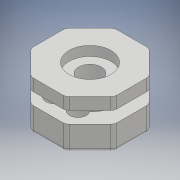
# Autodesk Inventor part: tendon anchor
Saved by Autodesk Inventor 2017 (Build 210142000, 142)
## iProperties
Created: 2018-09-01
Part Number: tendon anchor
Material: Generic
Document SubType Name: Modeling
Designer: jakub.tomczynski
Density: 1 g/cm^3
Appearance: Default
Author: jakub.tomczynski
## iProperties of the stored document tendon anchor_3DPrint.ipt
Created: 2018-09-01
Part Number: tendon anchor_3DPrint
Material: Generic
Document SubType Name: Modeling
Designer: jakub.tomczynski
Density: 1 g/cm^3
Appearance: Default
Author: jakub.tomczynski
Autodesk Inventor part; units mm, degrees
ref_plane "YZ Plane" through (0, 0, 0) normal (1, 0, 0) x (0, 1, 0)
ref_plane "XZ Plane" through (0, 0, 0) normal (0, 1, 0) x (-1, 0, 0)
sketch "Sketch1" plane through (0, 0, 0) normal (0, 0, 1) x (1, 0, 0)
  line L0 (1.4497, 3.5) -> (3.5, 1.4497)
  line L1 (3.5, 1.4497) -> (3.5, -1.4497)
  line L2 (3.5, -1.4497) -> (1.4497, -3.5)
  line L3 (1.4497, -3.5) -> (-1.4497, -3.5)
  line L4 (-1.4497, -3.5) -> (-3.5, -1.4497)
  line L5 (-3.5, -1.4497) -> (-3.5, 1.4497)
  line L6 (-3.5, 1.4497) -> (-1.4497, 3.5)
  line L7 (-1.4497, 3.5) -> (1.4497, 3.5)
  point P0 (0, 0)
  point P1 (0, 0)
  dimension "d0" = 7
  constraints: 16 end point, 1 coincident, 1 horizontal, 17 other
  measures "d0" distance between parallel lines of L3 L7
extrude "Extrusion1" add sketch "Sketch1" along normal blind 4
fillet "Fillet1" radius 0.5 8 edges at (1.4497, -3.5, 2) (3.5, -1.4497, 2) (3.5, 1.4497, 2) (1.4497, 3.5, 2) (-1.4497, 3.5, 2) (-3.5, 1.4497, 2) (-3.5, -1.4497, 2) (-1.4497, -3.5, 2)
ref_plane "Work Plane1" through (0, 0, 2) normal (0, 0, -1) x (-1, 0, 0)
sketch "Sketch2" plane through (0, 0, 2) normal (0, 0, -1) x (-1, 0, 0)
  circle A0 centre (0, 0) radius 2.25
  line L0 (-3.3536, 1.5962) -> (-1.5962, 3.3536) projected
  line L1 (-1.2426, 3.5) -> (1.2426, 3.5) projected
  line L2 (1.5962, 3.3536) -> (3.3536, 1.5962) projected
  line L3 (3.5, 1.2426) -> (3.5, -1.2426) projected
  line L4 (3.3536, -1.5962) -> (1.5962, -3.3536) projected
  line L5 (1.2426, -3.5) -> (-1.2426, -3.5) projected
  line L6 (-1.5962, -3.3536) -> (-3.3536, -1.5962) projected
  line L7 (-3.5, -1.2426) -> (-3.5, 1.2426) projected
  arc A1 (1.2426, -3.5) -> (1.5962, -3.3536) centre (1.2426, -3) ccw projected
  arc A2 (-1.5962, -3.3536) -> (-1.2426, -3.5) centre (-1.2426, -3) ccw projected
  arc A3 (-3.5, -1.2426) -> (-3.3536, -1.5962) centre (-3, -1.2426) ccw projected
  arc A4 (-3.3536, 1.5962) -> (-3.5, 1.2426) centre (-3, 1.2426) ccw projected
  arc A5 (-1.2426, 3.5) -> (-1.5962, 3.3536) centre (-1.2426, 3) ccw projected
  arc A6 (1.5962, 3.3536) -> (1.2426, 3.5) centre (1.2426, 3) ccw projected
  arc A7 (3.5, 1.2426) -> (3.3536, 1.5962) centre (3, 1.2426) ccw projected
  arc A8 (3.3536, -1.5962) -> (3.5, -1.2426) centre (3, -1.2426) ccw projected
  dimension "d4" = 4.5
  constraints: 1 centre point, 1 coincident
  measures "d4" diameter of A0
extrude "Extrusion2" cut sketch "Sketch2" against normal blind 1
sketch "Sketch4" plane through (0, 0, 4) normal (0, 0, 1) x (1, 0, 0)
  point P0 (0, 0)
  point P1 (0, 0)
  constraints: 1 coincident
hole "Hole1" at (0, 0, 4) direction (0, 0, -1) diameter 1.9 end through all counterbore diameter 3.5 counterbore depth 0.8
sketch "Sketch5" plane through (0, 0, 0) normal (0, 0, -1) x (-1, 0, 0)
  line L0 (0, 0) -> (0, -2.9696) construction
  point P0 (1, -2)
  point P1 (-1, -2)
  dimension "d17" = 2
  dimension "d18" = 2
  constraints: 2 end point, 1 symmetric about line, 1 vertical
  measures "d17" distance of point (-1, -2) point (1, -2)
  measures "d18" vertical distance of L0.start point (-1, -2)
hole "Hole2" at (-1, -2, 0) at (1, -2, 0) direction (0, 0, 1) diameter 1.4 depth 2.5 tip angle 118
sketch "Sketch6" plane through (0, 0, 0) normal (0, 0, -1) x (-1, 0, 0)
  circle A0 centre (1, -2) radius 0.7 projected
  circle A1 centre (-1, -2) radius 0.7 projected
  line L0 (1, -2.7) -> (-1, -2.7)
  line L1 (-1, -1.3) -> (1, -1.3)
  point P0 (0, 0)
  constraints: 4 end point, 4 point on circle, 3 tangent, 1 parallel
extrude "Extrusion4" cut sketch "Sketch6" against normal blind 0.75 contours A0 L0 A1 L1
fillet "Fillet2" radius 1 1 edges at (2.25, 0, 3)
fillet "Fillet3" radius 0.2 16 edges at (3.4619, -1.434, 0) (2.4749, -2.4749, 0) (1.434, -3.4619, 0) (0, -3.5, 0) (-1.434, -3.4619, 0) (-2.4749, -2.4749, 0) (-3.4619, -1.434, 0) (-3.5, 0, 0) (-3.4619, 1.434, 0) (-2.4749, 2.4749, 0) (-1.434, 3.4619, 0) (0, 3.5, 0) (1.434, 3.4619, 0) (2.4749, 2.4749, 0) (3.4619, 1.434, 0) (3.5, 0, 0)
body "Solid1"
